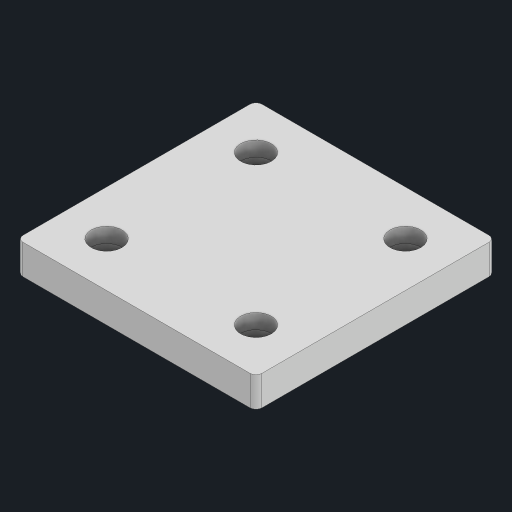
# Autodesk Inventor part: cradle_base
Saved by Autodesk Inventor 2024 (Build 280153000, 153)
## iProperties
Created: 2024-06-21
Part Number: cradle_base
Material: Generic
Document SubType Name: Modeling
Designer: mihir
Density: 1 g/cm^3
Appearance: Default
Author: mihir
Autodesk Inventor part; units mm, degrees
ref_plane "YZ Plane" through (0, 0, 0) normal (1, 0, 0) x (0, 1, 0)
ref_plane "XZ Plane" through (0, 0, 0) normal (0, 1, 0) x (-1, 0, 0)
ref_plane "XY Plane" through (0, 0, 0) normal (0, 0, 1) x (1, 0, 0)
sketch "Sketch1" plane through (0, 0, 0) normal (0, 1, 0) x (-1, 0, 0)
  line L0 (80, 0) -> (0, 0)
  line L1 (0, 0) -> (0, -80)
  line L2 (0, -80) -> (80, -80)
  line L3 (80, -80) -> (80, 0)
  dimension "d0" = 80
  constraints: 8 end point, 2 parallel, 2 perpendicular, 1 coincident, 1 horizontal
  measures "d0" distance of L2.end L0.start
extrude "Extrusion1" add sketch "Sketch1" along normal blind 10
sketch "Sketch2" plane through (0, 10, 0) normal (0, 1, 0) x (1, 0, 0)
  line L0 (-15, 15) -> (-65, 15) construction
  line L1 (-65, 15) -> (-65, 65) construction
  line L2 (-65, 65) -> (-15, 65) construction
  line L3 (-15, 65) -> (-15, 15) construction
  line L4 (-80, 0) -> (0, 0) construction
  line L5 (0, 0) -> (0, 80) construction
  dimension "d3" = 50
  dimension "d4" = 15
  dimension "d5" = 15
  constraints: 8 end point, 2 perpendicular, 2 vertical, 1 horizontal
  measures "d3" distance of L2.end L0.start
  measures "d4" distance from line of L4 L0.start
  measures "d5" distance from line of L5 L0.start
hole "Hole1" at (-15, 10, -15) at (-65, 10, -15) at (-15, 10, -65) at (-65, 10, -65) direction (0, -1, 0) diameter 6.3 depth 7.5 tip angle 118
sketch "Sketch3" plane through (0, 10, 0) normal (0, 1, 0) x (1, 0, 0)
  circle A0 centre (-65, 15) radius 3.15 projected
  circle A1 centre (-15, 15) radius 3.15 projected
  circle A2 centre (-65, 65) radius 3.15 projected
  circle A3 centre (-15, 65) radius 3.15 projected
  point P0 (0, 0)
  constraints: 4 coincident
hole "Hole2" at (-65, 10, -15) at (-15, 10, -15) at (-65, 10, -65) at (-15, 10, -65) direction (0, -1, 0) diameter 10.3 depth 5 tip angle 118
fillet "Fillet1" radius 2 4 edges at (-80, 5, 0) (0, 5, 0) (0, 5, -80) (-80, 5, -80)
equation "\"d0\" = base_width"
equation "\"d1\" = base_thickness"
equation "\"d3\" = rod_dist"
equation "\"d4\" = 0.5 * base_width - 0.5 * rod_dist"
equation "\"d5\" = 0.5 * base_width - 0.5 * rod_dist"
equation "\"d6\" = rod_tolerance + rod_diameter"
equation "\"d11\" = 0.75 * base_thickness"
equation "\"d13\" = rod_tolerance + post_diameter"
equation "\"d18\" = 0.5 * base_thickness"
equation "\"base_width\" = 80"
equation "\"base_thickness\" = 10"
equation "\"rod_diameter\" = 6"
equation "\"rod_tolerance\" = 0.3"
equation "\"post_diameter\" = 10"
equation "\"rod_dist\" = 50"
body "Solid1"
